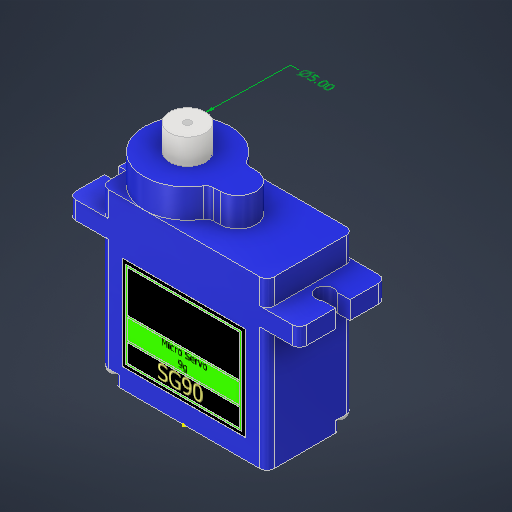
# Autodesk Inventor part: Part1_sG90
Saved by Autodesk Inventor 2026.2 (Build 302298010, 298A)
## iProperties
Created: 2025-10-06
Part Number: Part1_sG90
Material: Generic
Document SubType Name: Modeling
Designer: Zide
Density: 1 g/cm^3
Appearance: Default
Author: Zide
Autodesk Inventor part; units mm, degrees
ref_plane "YZ Plane" through (0, 0, 0) normal (1, 0, 0) x (0, 1, 0)
ref_plane "XZ Plane" through (0, 0, 0) normal (0, 1, 0) x (-1, 0, 0)
ref_plane "XY Plane" through (0, 0, 0) normal (0, 0, 1) x (1, 0, 0)
sketch "Sketch1" plane through (0, 0, 0) normal (0, 1, 0) x (-1, 0, 0)
  line L0 (10.5, 6) -> (-10.5, 6)
  line L1 (-11.5, 5) -> (-11.5, -5)
  line L2 (-10.5, -6) -> (10.5, -6)
  line L3 (11.5, -5) -> (11.5, 5)
  line L4 (11.5, 6) -> (-11.5, -6) construction
  line L5 (-11.5, 6) -> (11.5, -6) construction
  arc A0 (10.5, -6) -> (11.5, -5) centre (10.5, -5) ccw
  arc A1 (-11.5, -5) -> (-10.5, -6) centre (-10.5, -5) ccw
  arc A2 (-10.5, 6) -> (-11.5, 5) centre (-10.5, 5) ccw
  arc A3 (11.5, 5) -> (10.5, 6) centre (10.5, 5) ccw
  point P0 (0, 0)
  dimension "d0" = 23
  dimension "d1" = 12
  dimension "d2" = 1
  constraints: 12 end point, 8 point on circle, 8 point on line, 8 tangent, 4 centre point, 3 equal radius, 2 midpoint, 2 parallel, 1 horizontal, 1 perpendicular
  measures "d0" distance of L4.start L5.start
  measures "d1" distance of L4.end L5.start
  measures "d2" radius of A0
extrude "Extrusion1" add sketch "Sketch1" along normal blind 17
sketch "Sketch2" plane through (0, 0, 0) normal (0, -1, 0) x (1, 0, 0)
  arc A0 (-10.5, 6) -> (-11.5, 5) centre (-10.5, 5) ccw projected
  arc A1 (10.5, -6) -> (11.5, -5) centre (10.5, -5) ccw projected
  circle A2 centre (-10.5, 5) radius 1.125
  circle A3 centre (10.5, -5) radius 1.125
  point P0 (0, 0)
  dimension "d5" = 2.25
  dimension "d6" = 2.25
  constraints: 2 centre point, 1 coincident
  measures "d5" diameter of A2
  measures "d6" diameter of A3
extrude "Extrusion2" cut sketch "Sketch2" against normal blind 1.5
fillet "Fillet1" radius 0.5 4 edges at (9.9846, 0.75, -6) (11.5, 0.75, -4.4846) (-11.5, 0.75, 4.4846) (-9.9846, 0.75, 6)
sketch "Sketch3" plane through (0, 1.5, 0) normal (0, -1, 0) x (1, 0, 0)
  arc A0 (-10.5, 6) -> (-11.5, 5) centre (-10.5, 5) ccw projected
  arc A1 (-10.5, 6) -> (-10.5, 4) centre (-10.5, 5) ccw
  arc A2 (10.5, -4) -> (10.5, -6) centre (10.5, -5) ccw
  line L0 (10.5, -6) -> (10.5, -4)
  line L1 (-10.5, 4) -> (-10.5, 6)
  point P0 (0, 0)
  constraints: 4 end point, 4 point on circle, 2 centre point, 2 coincident, 2 vertical
revolve "Revolution1" add sketch "Sketch3" angle 180 about axis through (10.5, 1.5, -6) along (0, 0, 1) separate body contours L0 A2
revolve "Revolution2" add sketch "Sketch3" angle 180 about axis through (-10.5, 1.5, 4) along (0, 0, 1) separate body contours L1 A1 A0
sketch "Sketch5" plane through (0, 17, 0) normal (0, 1, 0) x (1, 0, 0)
  line L0 (16, 6) -> (-16, 6)
  line L1 (-16, -6) -> (16, -6)
  line L2 (16, -6) -> (-16, 6) construction
  line L3 (16, 6) -> (-16, -6) construction
  line L4 (10.5, 6) -> (-10.5, 6) projected
  arc A0 (-14.25, -1) -> (-14.25, 1) centre (-13.5, 0) ccw
  line L5 (-14.25, 1) -> (-16, 1)
  line L6 (-14.25, -1) -> (-16, -1)
  line L7 (-16, 6) -> (-16, 1)
  line L8 (-16, -1) -> (-16, -6)
  arc A1 (14.25, 1) -> (14.25, -1) centre (13.5, 0) ccw
  line L9 (14.25, 1) -> (16, 1)
  line L10 (14.25, -1) -> (16, -1)
  line L11 (16, -6) -> (16, -1)
  line L12 (16, 1) -> (16, 6)
  point P0 (0, 0)
  dimension "d22" = 32
  constraints: 24 end point, 5 parallel, 4 point on circle, 2 centre point, 2 horizontal, 2 midpoint, 2 perpendicular
  measures "d22" distance of L0.end L0.start
extrude "Extrusion3" add sketch "Sketch5" along normal blind 2.5 bodies 1
fillet "Fillet2" radius 1 4 edges at (16, 18.25, -6) (16, 18.25, 6) (-16, 18.25, 6) (-16, 18.25, -6)
sketch "Sketch6" plane through (0, 19.5, 0) normal (0, 1, 0) x (1, 0, 0)
  line L0 (-11.5, 5) -> (-11.5, -5) projected
  arc A0 (-11.5, -5) -> (-10.5, -6) centre (-10.5, -5) ccw projected
  arc A1 (-10.5, 6) -> (-11.5, 5) centre (-10.5, 5) ccw projected
  line L1 (11.5, -5) -> (11.5, 5) projected
  arc A2 (11.5, 5) -> (10.5, 6) centre (10.5, 5) ccw projected
  arc A3 (10.5, -6) -> (11.5, -5) centre (10.5, -5) ccw projected
  line L2 (-10.5, 6) -> (10.5, 6)
  line L3 (-10.5, -6) -> (-8.9538, -6) projected
  line L4 (-10.5, -6) -> (10.5, -6)
  point P0 (0, 0)
  constraints: 4 end point, 1 collinear, 1 tangent
extrude "Extrusion4" add sketch "Sketch6" along normal blind 3.5 bodies 1
sketch "Sketch7" plane through (0, 23, 0) normal (0, 1, 0) x (1, 0, 0)
  line L0 (-11.5, 5) -> (-11.5, -5) projected
  line L1 (-11.5, -3.4538) -> (-11.5, 5) projected
  line L2 (0, 0) -> (1.5, 0)
  arc A0 (1.5, -2.5) -> (1.5, 2.5) centre (1.5, 0) ccw
  line L3 (1.5, 2.5) -> (-0.0456, 2.5)
  line L4 (1.5, -2.5) -> (-0.0456, -2.5)
  arc A1 (-0.0456, 2.5) -> (-0.0456, -2.5) centre (-5.5, 0) ccw
  constraints: 6 end point, 4 point on circle, 3 horizontal, 2 centre point, 2 tangent, 1 coincident
extrude "Extrusion5" add sketch "Sketch7" along normal blind 4 bodies 1
fillet "Fillet3" radius 1 2 edges at (-0.0456, 25, 2.5) (-0.0456, 25, -2.5)
sketch "Sketch8" plane through (0, 27, 0) normal (0, 1, 0) x (1, 0, 0)
  arc A0 (-0.3038, 3) -> (-0.3038, -3) centre (-5.5, 0) ccw projected
  circle A1 centre (-5.5, 0) radius 0.5
  point P0 (0, 0)
  dimension "d38" = 1
  constraints: 1 centre point, 1 coincident
  measures "d38" diameter of A1
extrude "Extrusion6" add sketch "Sketch8" along normal blind 3.5 bodies 1
sketch "Sketch9" plane through (0, 27, 0) normal (0, 1, 0) x (1, 0, 0)
  circle A0 centre (-5.5, 0) radius 0.5 projected
  circle A1 centre (-5.5, 0) radius 2.5
  point P0 (0, 0)
  constraints: 1 centre point, 1 coincident
extrude "Extrusion7" add sketch "Sketch9" along normal blind 3.5 separate body
sketch "Sketch10" plane through (-8.9538, 0, 6) normal (0, 0, 1) x (1, 0, 0)
  line L0 (-1.5462, 1.5) -> (-1.5462, 17)
  line L1 (0.4538, 2.75) -> (17.4538, 2.75)
  line L2 (17.4538, 2.75) -> (17.4538, 15.75)
  line L3 (17.4538, 15.75) -> (0.4538, 15.75)
  line L4 (0.4538, 15.75) -> (0.4538, 2.75)
  line L5 (0.4538, 2.75) -> (17.4538, 15.75) construction
  line L6 (17.4538, 2.75) -> (0.4538, 15.75) construction
  point P0 (8.9538, 0)
  dimension "d44" = 17
  dimension "d45" = 13
  constraints: 14 end point, 2 parallel, 1 horizontal, 1 perpendicular
  measures "d44" distance of L1.start L1.end
  measures "d45" distance of L2.end L1.end
extrude "Extrusion8" add sketch "Sketch10" along normal blind 0.025 bodies 1
sketch "Sketch11" plane through (-8.9538, 0, 6.025) normal (0, 0, 1) x (1, 0, 0)
  line L0 (0.4538, 2.75) -> (17.4538, 2.75) projected
  line L1 (17.4538, 2.75) -> (17.4538, 15.75) projected
  line L2 (17.4538, 15.75) -> (0.4538, 15.75) projected
  line L3 (0.4538, 15.75) -> (0.4538, 2.75) projected
  line L4 (0.9538, 15.25) -> (16.9538, 15.25)
  line L5 (16.9538, 15.25) -> (16.9538, 3.25)
  line L6 (16.9538, 3.25) -> (0.9538, 3.25)
  line L7 (0.9538, 3.25) -> (0.9538, 15.25)
  line L8 (16.7038, 15) -> (1.2038, 15)
  line L9 (1.2038, 3.5) -> (16.7038, 3.5)
  line L10 (16.7038, 9.25) -> (1.2038, 9.25)
  line L11 (16.7038, 9) -> (1.2038, 9)
  line L12 (1.2038, 6.25) -> (16.7038, 6.25)
  line L13 (1.2038, 6) -> (16.7038, 6)
  line L14 (1.2038, 15) -> (1.2038, 9.25)
  line L15 (1.2038, 9) -> (1.2038, 6.25)
  line L16 (1.2038, 6) -> (1.2038, 3.5)
  line L17 (1.2038, 9) -> (1.2038, 6.25)
  line L18 (1.2038, 6) -> (1.2038, 3.5)
  line L19 (16.7038, 3.5) -> (16.7038, 6)
  line L20 (16.7038, 6.25) -> (16.7038, 9)
  line L21 (16.7038, 9.25) -> (16.7038, 15)
  point P0 (8.9538, 0)
  dimension "d48" = 0.5
  dimension "d49" = 0.25
  dimension "d50" = 0.25
  dimension "d51" = 0.25
  constraints: 36 end point, 5 perpendicular, 2 parallel, 3 other
  measures "d48" distance between parallel lines of L2 L4
  measures "d49" distance between parallel lines of L4 L8
  measures "d50" distance between parallel lines of L10 L11
  measures "d51" distance between parallel lines of L12 L13
extrude "Extrusion9" add sketch "Sketch11" along normal blind 0.025 contours L4 L5 L6 L7 bodies 1
sketch "Sketch12" plane through (-8.9538, 0, 6.025) normal (0, 0, 1) x (1, 0, 0)
  line L0 (5.8302, 8.978) -> (21.2508, 8.978) construction
  line L1 (21.2508, 8.978) -> (21.2508, 6.2497) construction
  line L2 (21.2508, 6.2497) -> (5.8302, 6.2497) construction
  line L3 (5.8302, 6.2497) -> (5.8302, 8.978) construction
  point P0 (8.9538, 0)
  constraints: 2 other
sketch "Sketch13" plane through (-8.9538, 0, 6.025) normal (0, 0, 1) x (1, 0, 0)
  line L0 (5.268, 5.8598) -> (20.7463, 5.8598) construction
  line L1 (20.7463, 5.8598) -> (20.7463, 3.3385) construction
  line L2 (20.7463, 3.3385) -> (5.268, 3.3385) construction
  line L3 (5.268, 3.3385) -> (5.268, 5.8598) construction
  point P0 (8.9538, 0)
  constraints: 2 other
body "Solid1"
body "Solid2"
body "Solid3"
body "Solid4"
